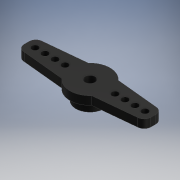
# Autodesk Inventor part: ServoArm2
Saved by Autodesk Inventor 2018.3 (Build 223284000, 284)
## iProperties
Created: 2020-03-24
Part Number: ServoArm2
Material: Generic
Document SubType Name: Modeling
Designer: Ivan
Density: 1 g/cm^3
Appearance: Default
Author: Ivan
Autodesk Inventor part; units mm, degrees
ref_plane "YZ Plane" through (0, 0, 0) normal (1, 0, 0) x (0, 1, 0)
ref_plane "XZ Plane" through (0, 0, 0) normal (0, 1, 0) x (-1, 0, 0)
ref_plane "XY Plane" through (0, 0, 0) normal (0, 0, 1) x (1, 0, 0)
sketch "Sketch1" plane through (0, 0, 0) normal (0, 0, 1) x (1, 0, 0)
  circle A0 centre (0, 0) radius 1.5
  circle A1 centre (0, 0) radius 6
  line L0 (-19, 2.75) -> (-1.5, 2.75)
  line L1 (-1.5, 2.75) -> (-1.5, -2.75)
  line L2 (-1.5, -2.75) -> (-19, -2.75)
  line L3 (-19, -2.75) -> (-19, 2.75)
  line L4 (0, -8.4) -> (0, 8.4) construction
  line L5 (19, 2.75) -> (1.5, 2.75)
  line L6 (1.5, 2.75) -> (1.5, -2.75)
  line L7 (1.5, -2.75) -> (19, -2.75)
  line L8 (19, -2.75) -> (19, 2.75)
  point P0 (-1.5, 0)
  dimension "d0" = 3
  dimension "d1" = 12
  dimension "d2" = 17.5
  dimension "d3" = 5.5
  constraints: 16 end point, 4 symmetric about line, 2 centre point, 2 coincident, 2 parallel, 1 horizontal, 1 horizontal alignment, 1 midpoint, 1 perpendicular, 1 tangent
  measures "d0" diameter of A0
  measures "d1" diameter of A1
  measures "d2" distance of L1.end L2.end
  measures "d3" distance between parallel lines of L0 L2
extrude "Extrusion1" add sketch "Sketch1" along normal blind 2.5 contours L6 L7 A1 L2 L1 A0 | A0 L1 L0 A1 L5 L6 | L6 L5 A1 L7 | L1 L2 A1 L0 | L5 L8 L7 A1 | A1 L2 L3 L0
fillet "Fillet1" radius 2 4 edges at (-19, 2.75, 1.25) (-19, -2.75, 1.25) (19, 2.75, 1.25) (19, -2.75, 1.25)
chamfer "Chamfer6" distance 11.6666 distance2 1.5 1 edges at (-5.3327, 2.75, 1.25) measured on face at (-13.1109, 2.75, 0.8333)
chamfer "Chamfer7" distance 11.6666 distance2 1.5 1 edges at (5.3327, 2.75, 1.25) measured on face at (13.1109, 2.75, 0.8333)
chamfer "Chamfer8" distance 11.6666 distance2 1.5 1 edges at (-5.3327, -2.75, 1.25) measured on face at (-9.2218, -2.75, 1.6667)
chamfer "Chamfer9" distance 11.6666 distance2 1.5 1 edges at (5.3327, -2.75, 1.25) measured on face at (9.2218, -2.75, 0.8333)
sketch "Sketch3" plane through (0, 0, 2.5) normal (0, 0, 1) x (1, 0, 0)
  circle A0 centre (-7.5, 0) radius 1
  line L0 (-26.6, 0) -> (26.6, 0) construction
  circle A1 centre (-10.5, 0) radius 1
  circle A2 centre (-13.5, 0) radius 1
  circle A3 centre (-16.5, 0) radius 1
  line L1 (0, -8.4) -> (0, 8.4) construction
  circle A4 centre (7.5, 0) radius 1
  circle A5 centre (10.5, 0) radius 1
  circle A6 centre (13.5, 0) radius 1
  circle A7 centre (16.5, 0) radius 1
  point P0 (0, 0)
  dimension "d37" = 2
  dimension "d38" = 7.5
  dimension "d41" = 3
  constraints: 8 centre point, 4 symmetric about line, 1 horizontal, 1 horizontal alignment, 10 other
  measures "d37" diameter of A0
  measures "d38" distance of A0.centre point (0, 0)
  measures "d41" distance of A0.centre A1.centre
extrude "Extrusion3" cut sketch "Sketch3" against normal through all
sketch "Sketch4" plane through (0, 0, 0) normal (0, 0, -1) x (-1, 0, 0)
  circle A0 centre (0, 0) radius 1.5 projected
  circle A1 centre (0, 0) radius 2.5
  circle A2 centre (0, 0) radius 4.25
  dimension "d48" = 5
  dimension "d49" = 8.5
  constraints: 2 centre point, 2 coincident
  measures "d48" diameter of A1
  measures "d49" diameter of A2
extrude "Extrusion4" add sketch "Sketch4" along normal blind 3 contours A2
body "Solid1"
